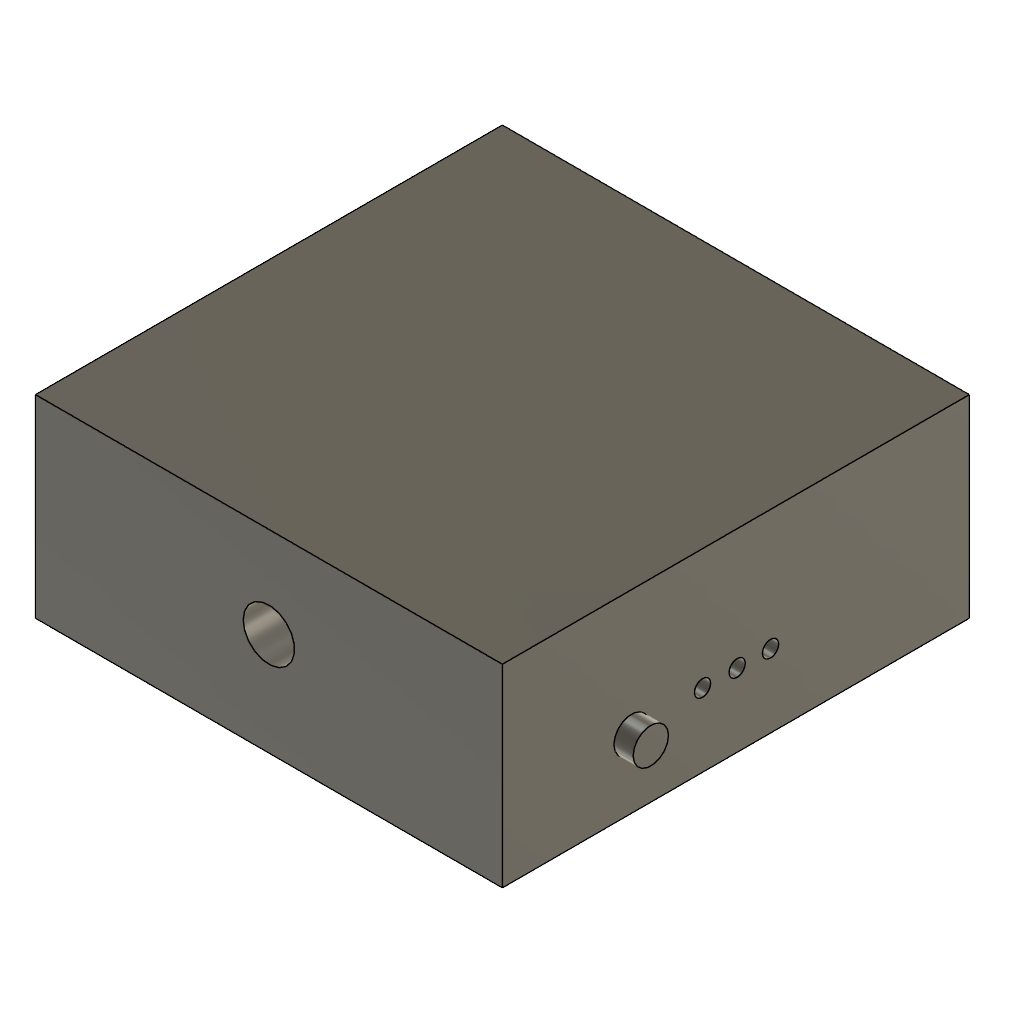
VTX_Envelope (Autodesk Fusion 360 design; units mm, degrees)
part number: 2026-09-21-19-44-39-891
Autodesk Fusion 360 part; units mm, degrees
sketch "Sketch1" plane through (0, 0, 0) normal (0, 0, 1) x (1, 0, 0)
  line L0 (-18.2, 18.2) -> (18.2, 18.2)
  line L1 (18.2, 18.2) -> (18.2, -18.2)
  line L2 (18.2, -18.2) -> (-18.2, -18.2)
  line L3 (-18.2, -18.2) -> (-18.2, 18.2)
  line L4 (-18.2, 18.2) -> (18.2, -18.2) construction
  line L5 (18.2, 18.2) -> (-18.2, -18.2) construction
  dimension "d1" = 36.4
  dimension "d2" = 36.4
  constraint horizontal L0
  constraint perpendicular L0 L1
  constraint parallel L0 L2
  constraint parallel L1 L3
  constraint coincident L4 origin
  constraint coincident L5 origin
  measures "d1" distance of L0.end L1.end
  measures "d2" distance of L1.end L2.end
extrude "Extrude1" add sketch "Sketch1" along normal blind 15.1
sketch "Sketch2" plane through (0, 0, 0) normal (0, 0, -1) x (1, 0, 0)
  line L0 (18.2, 18.2) -> (-18.2, 18.2)
  line L1 (-18.2, 18.2) -> (-18.2, -18.2)
  line L2 (-18.2, -18.2) -> (18.2, -18.2)
  line L3 (18.2, -18.2) -> (18.2, 18.2)
  circle A0 centre (-10, 10) radius 1
  circle A1 centre (10, 10) radius 1
  circle A2 centre (10, -10) radius 1
  circle A3 centre (-10, -10) radius 1
  dimension "d5" = 2
  dimension "d6" = 2
  dimension "d7" = 2
  dimension "d8" = 2
  dimension "d9" = 10
  dimension "d10" = 10
  dimension "d11" = 10
  dimension "d12" = 10
  dimension "d13" = 10
  dimension "d14" = 10
  dimension "d15" = 10
  dimension "d16" = 10
  measures "d5" diameter of A0
  measures "d6" diameter of A1
  measures "d7" diameter of A2
  measures "d8" diameter of A3
  measures "d9" horizontal distance of origin A0.centre
  measures "d10" vertical distance of origin A0.centre
  measures "d11" vertical distance of origin A2.centre
  measures "d12" horizontal distance of origin A2.centre
  measures "d13" vertical distance of origin A1.centre
  measures "d14" horizontal distance of origin A1.centre
  measures "d15" vertical distance of origin A3.centre
  measures "d16" horizontal distance of origin A3.centre
sketch "Sketch3" plane through (0, -18.2, 0) normal (0, -1, 0) x (1, 0, 0)
  line L0 (-18.2, 0) -> (18.2, 0)
  line L1 (18.2, 0) -> (18.2, 15.1)
  line L2 (18.2, 15.1) -> (-18.2, 15.1)
  line L3 (-18.2, 15.1) -> (-18.2, 0)
  line L4 (-5.0331, 11.4393) -> (4.9669, 11.4393)
  line L5 (4.9669, 11.4393) -> (4.9669, 3.4393)
  line L6 (4.9669, 3.4393) -> (-5.0331, 3.4393)
  line L7 (-5.0331, 3.4393) -> (-5.0331, 11.4393)
  dimension "d17" = 10
  dimension "d18" = 8
  constraint horizontal L4
  constraint vertical L5
  constraint horizontal L6
  constraint vertical L7
  measures "d17" distance of L4.start L4.end
  measures "d18" distance of L4.start L6.end
extrude "Extrude2" add sketch "Sketch3" along normal blind 3 contours L4 L5 L6 L7
sketch "Sketch4" plane through (18.2, 0, 0) normal (1, 0, 0) x (0, 1, 0)
  line L0 (-18.2, 0) -> (18.2, 0)
  line L1 (18.2, 0) -> (18.2, 15.1)
  line L2 (18.2, 15.1) -> (-18.2, 15.1)
  line L3 (-18.2, 15.1) -> (-18.2, 0)
  line L4 (-9.8702, 10.5872) -> (10.1298, 10.5872)
  line L5 (10.1298, 10.5872) -> (10.1298, 4.5872)
  line L6 (10.1298, 4.5872) -> (-9.8702, 4.5872)
  line L7 (-9.8702, 4.5872) -> (-9.8702, 10.5872)
  dimension "d21" = 20
  dimension "d22" = 6
  constraint horizontal L4
  constraint vertical L5
  constraint horizontal L6
  constraint vertical L7
  measures "d21" distance of L4.start L4.end
  measures "d22" distance of L4.start L6.end
extrude "Extrude3" add sketch "Sketch4" along normal blind 3 contours L4 L5 L6 L7
sketch "Sketch5" plane through (0, 18.2, 0) normal (0, 1, 0) x (-1, 0, 0)
  line L0 (-18.2, 0) -> (18.2, 0)
  line L1 (18.2, 0) -> (18.2, 15.1)
  line L2 (18.2, 15.1) -> (-18.2, 15.1)
  line L3 (-18.2, 15.1) -> (-18.2, 0)
  line L4 (-5.1038, 11.5152) -> (4.8962, 11.5152)
  line L5 (4.8962, 11.5152) -> (4.8962, 3.5152)
  line L6 (4.8962, 3.5152) -> (-5.1038, 3.5152)
  line L7 (-5.1038, 3.5152) -> (-5.1038, 11.5152)
  dimension "d25" = 10
  dimension "d26" = 8
  constraint horizontal L4
  constraint vertical L5
  constraint horizontal L6
  constraint vertical L7
  measures "d25" distance of L4.start L4.end
  measures "d26" distance of L4.start L6.end
extrude "Extrude4" add sketch "Sketch5" along normal blind 3 contours L4 L5 L6 L7
move_face "MoveFace1" by (0, 3, 0) 1 faces at (-1.6998, -21.2, 8.7727)
sketch "Sketch6" plane through (0, -18.2, 0) normal (0, -1, 0) x (1, 0, 0)
  line L0 (-18.2, 0) -> (18.2, 0)
  line L1 (18.2, 0) -> (18.2, 15.1)
  line L2 (18.2, 15.1) -> (-18.2, 15.1)
  line L3 (-18.2, 15.1) -> (-18.2, 0)
  circle A0 centre (0, 8) radius 2
  dimension "d29" = 4
  measures "d29" diameter of A0
extrude "Extrude5" cut sketch "Sketch6" against normal blind 3 contours A0
move_face "MoveFace2" by (0, -3, 0) 1 faces at (-1.5629, 21.2, 6.1819)
sketch "Sketch7" plane through (0, 18.2, 0) normal (0, 1, 0) x (-1, 0, 0)
  line L0 (-18.2, 0) -> (18.2, 0)
  line L1 (18.2, 0) -> (18.2, 15.1)
  line L2 (18.2, 15.1) -> (-18.2, 15.1)
  line L3 (-18.2, 15.1) -> (-18.2, 0)
  line L4 (-2.9909, 1.0739) -> (4.5091, 1.0739)
  line L5 (4.5091, 1.0739) -> (4.5091, 5.0739)
  line L6 (4.5091, 5.0739) -> (-2.9909, 5.0739)
  line L7 (-2.9909, 5.0739) -> (-2.9909, 1.0739)
  dimension "d32" = 7.5
  dimension "d33" = 4
  constraint horizontal L4
  constraint vertical L5
  constraint horizontal L6
  constraint vertical L7
  measures "d32" distance of L4.start L4.end
  measures "d33" distance of L4.start L6.end
extrude "Extrude6" cut sketch "Sketch7" against normal blind 4 contours L4 L5 L6 L7
move_face "MoveFace3" by (-3, 0, 0) 1 faces at (21.2, -3.2035, 8.5872)
sketch "Sketch8" plane through (18.2, 0, 0) normal (1, 0, 0) x (0, 1, 0)
  line L0 (-18.2, 0) -> (18.2, 0)
  line L1 (18.2, 0) -> (18.2, 15.1)
  line L2 (18.2, 15.1) -> (-18.2, 15.1)
  line L3 (-18.2, 15.1) -> (-18.2, 0)
  circle A0 centre (-8.1313, 5.3193) radius 1.3754
extrude "Extrude7" add sketch "Sketch8" along normal blind 1.5 contours A0
sketch "Sketch9" plane through (18.2, 0, 0) normal (1, 0, 0) x (0, 1, 0)
  circle A0 centre (-8.1313, 5.3193) radius 1.3754
  line L0 (-18.2, 0) -> (18.2, 0)
  line L1 (18.2, 0) -> (18.2, 15.1)
  line L2 (18.2, 15.1) -> (-18.2, 15.1)
  line L3 (-18.2, 15.1) -> (-18.2, 0)
  circle A1 centre (-2.6, 5.7) radius 0.6325
  circle A2 centre (0.1, 5.7) radius 0.6325
  circle A3 centre (2.7, 5.7) radius 0.6325
  dimension "d38" = 1.265
  dimension "d39" = 1.265
  measures "d38" diameter of A2
  measures "d39" diameter of A3
extrude "Extrude8" cut sketch "Sketch9" against normal blind 1.4 contours A1 | A2 | A3
extrude "Extrude9" cut sketch "Sketch2" against normal blind 3 contours A0 | A1 | A2 | A3
named bodies: "VTX_body"
